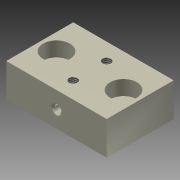
# Autodesk Inventor part: 13_0204_073
Saved by Autodesk Inventor 2012 SP1 (Build 160190100, 190)
## iProperties
Created: 2013-05-07
Part Number: 13_0204_073
Material: Default
Document SubType Name: Modeling
Designer: vogel
Density: 1 g/cm^3
Author: vogel
Autodesk Inventor part; units mm, degrees
ref_plane "YZ Plane" through (0, 0, 0) normal (1, 0, 0) x (0, 1, 0)
ref_plane "XZ Plane" through (0, 0, 0) normal (0, 1, 0) x (-1, 0, 0)
ref_plane "XY Plane" through (0, 0, 0) normal (0, 0, 1) x (1, 0, 0)
sketch "Skizze1" plane through (0, 0, 0) normal (0, 0, 1) x (1, 0, 0)
  line L0 (0, 0) -> (30, 0)
  line L1 (30, 0) -> (30, 20)
  line L2 (30, 20) -> (0, 20)
  line L3 (0, 20) -> (0, 0)
  dimension "d0" = 20
  dimension "d1" = 30
  constraints: 8 end point, 2 parallel, 1 horizontal, 1 perpendicular
  measures "d0" distance of L2.end L0.start
  measures "d1" distance of L0.start L0.end
extrude "Extrusion1" add sketch "Skizze1" along normal blind 10
sketch "Skizze2" plane through (0, 0, 10) normal (0, 0, 1) x (1, 0, 0)
  line L0 (0, 0) -> (0, 20) projected
  line L1 (30, 0) -> (0, 0) projected
  line L2 (30, 20) -> (30, 0) projected
  line L3 (0, 20) -> (30, 20) projected
  line L4 (0, 10) -> (30, 10)
  line L5 (15, 20) -> (15, 0)
  point P0 (5, 10)
  point P1 (25, 10)
  dimension "d4" = 20
  constraints: 4 end point, 4 midpoint, 2 point on line, 1 symmetric about line
  measures "d4" distance of point (25, 10) point (5, 10)
hole "Bohrung1" at (5, 10, 10) at (25, 10, 10) direction (0, 0, -1) diameter 4.5 end through all counterbore diameter 8 counterbore depth 4.4
sketch "Skizze3" plane through (0, 0, 10) normal (0, 0, 1) x (1, 0, 0)
  circle A0 centre (25, 10) radius 4 projected
  circle A1 centre (5, 10) radius 4 projected
  line L0 (30, 0) -> (0, 0) projected
  line L1 (0, 20) -> (30, 20) projected
  line L2 (15, 20) -> (15, 0)
  line L3 (5, 10) -> (25, 10)
  point P0 (15, 15)
  point P1 (15, 5)
  dimension "d12" = 10
  constraints: 4 end point, 2 midpoint, 2 point on line, 1 perpendicular, 1 symmetric about line
  measures "d12" distance of point (15, 5) point (15, 15)
hole "Bohrung2" at (15, 15, 10) at (15, 5, 10) direction (0, 0, -1) diameter 2.459 end through all thread size "M3x0.5" class "6H" standard "ISO Metric profile"
sketch "Skizze4" plane through (0, 20, 0) normal (0, 1, 0) x (1, 0, 0)
  line L0 (0, -10) -> (30, -10) projected
  line L1 (30, 0) -> (0, 0) projected
  line L2 (15, 0) -> (15, -10)
  point P0 (15, -5)
  dimension "d20" = 5
  constraints: 3 midpoint, 2 end point
  measures "d20" distance from line of L1 point (15, -5)
hole "Bohrung3" at (15, 20, 5) direction (0, -1, 0) diameter 2 end through all
chamfer "Fase1" distance 0.5 angle 45 2 edges at (15, 20, 4) (15, 0, 4)
sketch "Skizze5" plane through (0, 0, 0) normal (0, -1, 0) x (1, 0, 0)
  line L0 (30, 10) -> (0, 10) projected
  line L1 (0, 0) -> (0, 10) projected
  line L2 (0, 0) -> (30, 0) projected
  line L3 (7.5, 10) -> (22.5, 10)
  line L4 (22.5, 10) -> (22.5, 0)
  line L5 (22.5, 0) -> (7.5, 0)
  line L6 (7.5, 0) -> (7.5, 10)
  line L7 (15, 10) -> (15, 0)
  dimension "d31" = 15
  dimension "d32" = 15
  constraints: 10 end point, 2 midpoint, 2 parallel, 2 perpendicular, 2 point on line, 1 horizontal, 1 other
  measures "d31" distance between parallel lines of L1 L7
  measures "d32" distance between parallel lines of L4 L6
extrude "Extrusion2" cut sketch "Skizze5" against normal blind 3 contours L4 L2 L7 L0 | L7 L2 L6 L0
